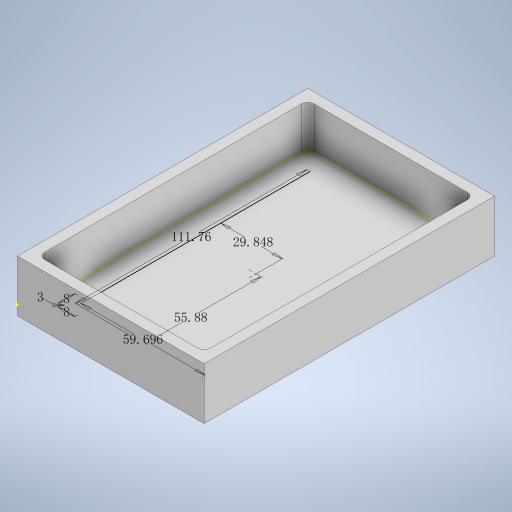
# Autodesk Inventor part: PrismGC
Saved by Autodesk Inventor 2024 (Build 280153000, 153)
## iProperties
Created: 2023-08-08
Part Number: PrismGC
Material: 常规
Document SubType Name: Modeling
Designer: liyuxuan
Density: 1 g/cm^3
Appearance: 默认
Author: liyuxuan
Autodesk Inventor part; units mm, degrees
ref_plane "YZ Plane" through (0, 0, 0) normal (1, 0, 0) x (0, 1, 0)
ref_plane "XZ Plane" through (0, 0, 0) normal (0, 1, 0) x (-1, 0, 0)
ref_plane "XY Plane" through (0, 0, 0) normal (0, 0, 1) x (1, 0, 0)
sketch "草图1" plane through (0, 0, 0) normal (0, 1, 0) x (-1, 0, 0)
  line L0 (0, 0) -> (-90, 0)
  line L1 (-90, 0) -> (-90, -140)
  line L2 (-90, -140) -> (0, -140)
  line L3 (0, -140) -> (0, 0)
  dimension "d0" = 140
  dimension "d1" = 90
  constraints: 8 end point, 2 parallel, 1 horizontal, 1 perpendicular
  measures "d0" distance of L0.end L1.end
  measures "d1" distance of L1.end L2.end
extrude "拉伸1" add sketch "草图1" along normal blind 25
sketch "草图2" plane through (0, 25, 0) normal (0, 1, 0) x (1, 0, 0)
  line L0 (90, 0) -> (90, 140) projected
  line L1 (90, 140) -> (0, 140) projected
  line L2 (0, 140) -> (0, 0) projected
  line L3 (0, 0) -> (90, 0) projected
  line L4 (5, 5) -> (85, 5)
  line L5 (85, 5) -> (85, 135)
  line L6 (85, 135) -> (5, 135)
  line L7 (5, 135) -> (5, 5)
  line L8 (5, 5) -> (85, 135) construction
  line L9 (85, 5) -> (5, 135) construction
  point P0 (45, 70)
  dimension "d4" = 80
  dimension "d5" = 130
  constraints: 12 end point, 2 midpoint, 2 parallel, 1 horizontal, 1 perpendicular
  measures "d4" distance of L6.end L5.end
  measures "d5" distance of L5.end L4.end
extrude "拉伸2" cut sketch "草图2" against normal blind 20 contours L7 L6 L5 L4
fillet "面圆角1" radius 3 1 edges at (5, 15, -5)
fillet "面圆角2" radius 3 1 edges at (5, 15, -135)
fillet "面圆角3" radius 3 1 edges at (85, 15, -135)
fillet "面圆角4" radius 3 1 edges at (85, 15, -5)
sketch "草图4" plane through (0, 5, 0) normal (0, 1, 0) x (1, 0, 0)
  arc A0 (82, 5) -> (85, 8) centre (82, 8) ccw projected
  line L0 (85, 132) -> (85, 8) projected
  arc A1 (85, 132) -> (82, 135) centre (82, 132) ccw projected
  line L1 (8, 135) -> (82, 135) projected
  arc A2 (8, 135) -> (5, 132) centre (8, 132) ccw projected
  line L2 (5, 8) -> (5, 132) projected
  arc A3 (5, 8) -> (8, 5) centre (8, 8) ccw projected
  line L3 (82, 5) -> (8, 5) projected
  line L4 (16.152, 18.12) -> (14.152, 18.12)
  line L5 (11.152, 15.12) -> (11.152, 13.12)
  line L6 (14.152, 10.12) -> (16.152, 10.12)
  line L7 (19.152, 13.12) -> (19.152, 15.12)
  line L8 (19.152, 18.12) -> (11.152, 10.12) construction
  line L9 (11.152, 18.12) -> (19.152, 10.12) construction
  arc A4 (11.152, 13.12) -> (14.152, 10.12) centre (14.152, 13.12) ccw
  arc A5 (16.152, 10.12) -> (19.152, 13.12) centre (16.152, 13.12) ccw
  arc A6 (19.152, 15.12) -> (16.152, 18.12) centre (16.152, 15.12) ccw
  arc A7 (14.152, 18.12) -> (11.152, 15.12) centre (14.152, 15.12) ccw
  line L10 (15.152, 14.12) -> (74.848, 14.12)
  line L11 (15.152, 14.12) -> (15.152, 125.88)
  point P0 (0, 0)
  point P1 (45, 70)
  point P2 (45, 70)
  dimension "d12" = 55.88
  dimension "d13" = 29.848
  dimension "d14" = 8
  dimension "d15" = 8
  dimension "d16" = 3
  dimension "d17" = 59.696
  dimension "d18" = 111.76
  constraints: 16 end point, 8 point on circle, 8 point on line, 8 tangent, 4 centre point, 3 equal radius, 2 horizontal, 2 midpoint, 2 parallel, 2 perpendicular, 1 coincident, 1 other
  measures "d12" vertical distance of L10.start point (45, 70)
  measures "d13" horizontal distance of point (45, 70) L10.start
  measures "d14" distance of L9.end L8.end
  measures "d15" distance of L8.end L9.start
  measures "d16" radius of A4
  measures "d17" distance of L10.start L10.end
  measures "d18" distance of L10.start L11.end
